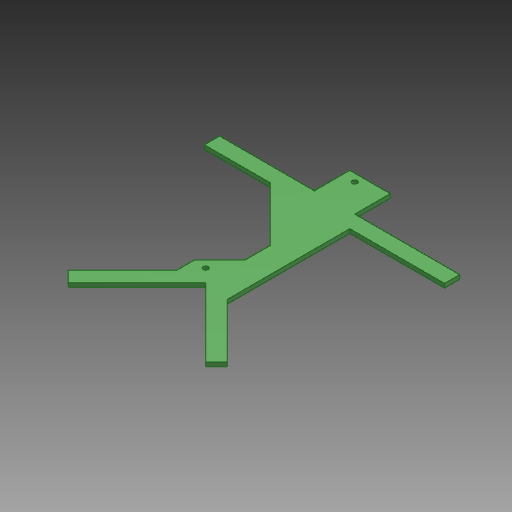
# Autodesk Inventor part: Color Detect PCB
Saved by Autodesk Inventor 2019.4 (Build 234330000, 330)
## iProperties
Part Number: Color Detect PCB
Material: Phenolharz
Document SubType Name: Modeling
Designer: rYan
Density: 1.38 g/cm^3
Appearance: Glatt - waldgrün
Mass: 4.46277 g
Surface Area: 47.9657 cm^2
Volume: 3.23389 cm^3
Author: rYan
Autodesk Inventor part; units mm, degrees
ref_plane "YZ Plane" through (0, 0, 0) normal (1, 0, 0) x (0, 1, 0)
ref_plane "XZ Plane" through (0, 0, 0) normal (0, 1, 0) x (-1, 0, 0)
ref_plane "XY Plane" through (0, 0, 0) normal (0, 0, 1) x (1, 0, 0)
sketch "Skizze1" plane through (0, 0, 0) normal (0, 0, 1) x (1, 0, 0)
  circle A0 centre (-57.772, 35) radius 20 construction
  circle A1 centre (57.772, 35) radius 20 construction
  circle A2 centre (35, -57.772) radius 20 construction
  circle A3 centre (-35, -57.772) radius 20 construction
  line L0 (0, 81.5544) -> (0, -104.3264) construction
  line L1 (-108.8808, 0) -> (108.8808, 0) construction
  circle A4 centre (0, 0) radius 25 construction
  line L2 (10, 25) -> (10, -23.5147)
  circle A5 centre (-6, -2.5) radius 6 construction
  line L3 (0, 3.5) -> (-21.5, 25)
  line L4 (0, -6.5) -> (-10, -16.5)
  line L5 (-10, -16.5) -> (-10, -23.5147)
  line L6 (-10, -23.5147) -> (-31.444, -44.9587)
  line L7 (-31.444, -44.9587) -> (-27.2013, -49.2013)
  line L8 (-27.2013, -49.2013) -> (0, -22)
  line L9 (0, -22) -> (27.2013, -49.2013)
  line L10 (27.2013, -49.2013) -> (31.444, -44.9587)
  line L11 (31.444, -44.9587) -> (10, -23.5147)
  line L12 (0, -6.5) -> (0, 3.5)
  line L13 (10, 25) -> (47.5055, 25)
  line L14 (47.5055, 25) -> (47.5055, 31)
  line L15 (-10, 31) -> (-47.5055, 31)
  line L16 (-47.5055, 31) -> (-47.5055, 25)
  line L17 (-47.5055, 25) -> (-21.5, 25)
  line L18 (-10, 31) -> (-10, 45)
  line L19 (-10, 45) -> (6, 45)
  line L20 (6, 45) -> (6, 31)
  line L21 (6, 31) -> (47.5055, 31)
  line L22 (-61.4468, -24.6516) -> (-51.4468, -24.6516) construction
  line L23 (-51.4468, -24.6516) -> (-56.4468, -27.5384) construction
  line L24 (-56.4468, -27.5384) -> (-61.4468, -24.6516) construction
  line L25 (-56.4468, -27.5384) -> (-56.4468, -24.6516) construction
  circle A6 centre (-27.2013, -44.9587) radius 3 construction
  circle A7 centre (-27.2013, -44.9587) radius 5 construction
  circle A8 centre (-44.5055, 28) radius 3 construction
  circle A9 centre (-44.5055, 28) radius 5 construction
  circle A10 centre (-5, -17) radius 1.05
  circle A11 centre (-5, 42) radius 1.05
  dimension "d0" = 35
  dimension "d1" = 57.772
  dimension "d2" = 40
  dimension "d3" = 57.772
  dimension "d4" = 35
  dimension "d5" = 40
  dimension "d6" = 50
  dimension "d7" = 10
  dimension "d9" = 6
  dimension "d10" = 2.5
  dimension "d11" = 12
  dimension "d12" = 6
  dimension "d13" = 6
  dimension "d14" = 4
  dimension "d15" = 10
  dimension "d16" = 6
  dimension "d20" = 31
  dimension "d21" = 10
  dimension "d22" = 120
  dimension "d23" = 2.8868
  dimension "d24" = 10
  dimension "d25" = 10
  dimension "d26" = 22
  dimension "d27" = 2.1
  dimension "d28" = 5
  dimension "d29" = 17
  dimension "d30" = 5
  dimension "d31" = 42
  dimension "d32" = 45
  dimension "d33" = 6
  constraints: 48 end point, 13 perpendicular, 12 centre point, 8 tangent, 4 collinear, 3 coincident, 3 point on line, 3 vertical, 2 horizontal, 2 parallel, 1 equal radius, 1 midpoint, 7 other
  measures "d0" distance from line of A1.centre L1
  measures "d1" distance from line of L0 A1.centre
  measures "d2" diameter of A1
  measures "d3" distance from line of A2.centre L1
  measures "d4" distance from line of A2.centre L0
  measures "d5" diameter of A2
  measures "d6" diameter of A4
  measures "d7" distance between parallel lines of L0 L2
  measures "d9" distance from line of A5.centre L0
  measures "d10" distance from line of A5.centre L1
  measures "d11" diameter of A5
  measures "d12" distance of L13.end L14.end
  measures "d13" horizontal distance of L3.start A5.centre
  measures "d14" vertical distance of L4.start A5.centre
  measures "d15" distance between parallel lines of L5 L0
  measures "d16" distance of L9.end L10.end
  measures "d20" distance between parallel lines of L1 L21
  measures "d21" distance of L22.start L22.end
  measures "d22" angle of L24 L23
  measures "d23" distance of L23.end L25.end
  measures "d24" diameter of A7
  measures "d25" diameter of A9
  measures "d26" distance from line of L1 L8.end
  measures "d27" diameter of A10
  measures "d28" distance from line of A10.centre L0
  measures "d29" distance from line of A10.centre L1
  measures "d30" distance from line of L0 A11.centre
  measures "d31" distance from line of A11.centre L1
  measures "d32" distance between parallel lines of L1 L19
  measures "d33" distance between parallel lines of L0 L20
extrude "Extrusion1" add sketch "Skizze1" along normal blind 1.6
equation "\"d3\" = d1"
equation "\"d4\" = d0"
equation "\"d5\" = d2"
equation "\"d25\" = d24"
